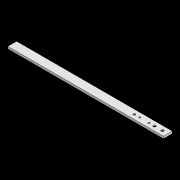
# Autodesk Inventor part: arm1_L
Saved by Autodesk Inventor 2022 (Build 260153000, 153)
## iProperties
Created: 2021-06-08
Part Number: arm1_L
Material: 一般
Document SubType Name: Modeling
Designer: yossy
Density: 1 g/cm^3
Appearance: 既定
Mass: 42.0818 g
Surface Area: 203.017 cm^2
Volume: 15.5858 cm^3
Author: yossy
Autodesk Inventor part; units mm, degrees
ref_plane "YZ Plane" through (0, 0, 0) normal (1, 0, 0) x (0, 1, 0)
ref_plane "XZ Plane" through (0, 0, 0) normal (0, 1, 0) x (-1, 0, 0)
ref_plane "XY Plane" through (0, 0, 0) normal (0, 0, 1) x (1, 0, 0)
sketch "スケッチ1" plane through (0, 0, 0) normal (0, 0, 1) x (1, 0, 0)
  line L0 (0, 0) -> (352, 0)
  line L1 (352, 0) -> (352, 5)
  line L2 (352, 5) -> (0, 5)
  line L3 (0, 5) -> (0, 0)
  line L4 (0, 0) -> (6, 0)
  line L5 (0, 1) -> (0, 0)
  dimension "d0" = 352
  dimension "d1" = 5
  constraints: 12 end point, 2 horizontal, 2 parallel, 1 perpendicular
  measures "d0" distance of L2.end L1.end
  measures "d1" distance of L1.end L0.end
extrude "押し出し1" add sketch "スケッチ1" along normal blind 20
sketch "スケッチ3" plane through (0, 0, 0) normal (-1, 0, 0) x (0, 0, 1)
  line L0 (0, 5) -> (0, 0) projected
  line L1 (0, 0) -> (20, 0) projected
  line L2 (20, 5) -> (20, 0) projected
  line L3 (0, 5) -> (20, 5) projected
  circle A0 centre (4, 2) radius 1.2
  circle A1 centre (16, 3) radius 1.2
  dimension "d14" = 2.4
  dimension "d15" = 2.4
  dimension "d16" = 3
  dimension "d17" = 4
  dimension "d18" = 4
  dimension "d19" = 3
  constraints: 2 centre point
  measures "d14" diameter of A0
  measures "d15" diameter of A1
  measures "d16" distance from line of L1 A1.centre
  measures "d17" distance from line of L2 A1.centre
  measures "d18" distance from line of L0 A0.centre
  measures "d19" distance from line of L3 A0.centre
extrude "押し出し3" cut sketch "スケッチ3" against normal blind 6 contours A0 | A1
sketch "スケッチ4" plane through (0, 0, 0) normal (0, -1, 0) x (1, 0, 0)
  line L0 (0, 0) -> (352, 0) projected
  line L1 (352, 0) -> (352, 20) projected
  line L2 (0, 20) -> (352, 20) projected
  line L3 (0, 0) -> (0, 20) projected
  line L4 (2, 2) -> (350, 2)
  line L5 (350, 2) -> (350, 18)
  line L6 (350, 18) -> (2, 18)
  line L7 (2, 18) -> (2, 2)
  dimension "d22" = 2
  dimension "d23" = 2
  dimension "d24" = 2
  dimension "d25" = 2
  constraints: 8 end point, 2 parallel, 1 horizontal, 1 perpendicular
  measures "d22" distance between parallel lines of L3 L7
  measures "d23" distance between parallel lines of L2 L6
  measures "d24" distance between parallel lines of L0 L4
  measures "d25" distance between parallel lines of L1 L5
extrude "押し出し4" cut sketch "スケッチ4" against normal blind 3 contours L7 L6 L5 L4
sketch "スケッチ6" plane through (0, 3, 0) normal (0, -1, 0) x (1, 0, 0)
  line L0 (350, 18) -> (350, 2) projected
  line L1 (2, 18) -> (350, 18) projected
  point P0 (0, 0)
  point P1 (340, 10)
  dimension "d35" = 10
  dimension "d36" = 8
  dimension "d37" = 16
  measures "d35" distance from line of L0 point (340, 10)
  measures "d36" distance from line of L1 point (340, 10)
  measures "d37" distance of L0.start L0.end
hole "穴1" at (340, 3, 10) direction (0, 1, 0) diameter 10 end through all
sketch "スケッチ7" plane through (0, 3, 0) normal (0, -1, 0) x (1, 0, 0)
  circle A0 centre (340, 10) radius 5 projected
  line L0 (340, 10) -> (322, 10)
  point P0 (0, 0)
  dimension "d38" = 18
  constraints: 2 end point, 1 horizontal
  measures "d38" distance of L0.start L0.end
hole "穴2" at (322, 3, 10) direction (0, 1, 0) diameter 6 end through all
sketch "スケッチ8" plane through (0, 3, 0) normal (0, -1, 0) x (1, 0, 0)
  circle A0 centre (322, 10) radius 3 projected
  line L0 (322, 10) -> (309.5, 10)
  point P0 (0, 0)
  dimension "d46" = 12.5
  constraints: 2 end point, 1 horizontal
  measures "d46" distance of L0.start L0.end
hole "穴3" at (309.5, 3, 10) direction (0, 1, 0) diameter 7 end through all
sketch "スケッチ9" plane through (0, 3, 0) normal (0, -1, 0) x (1, 0, 0)
  circle A0 centre (309.5, 10) radius 3.5 projected
  line L0 (309.5, 10) -> (288.5, 10)
  point P0 (0, 0)
  dimension "d54" = 21
  constraints: 2 end point, 1 horizontal
  measures "d54" distance of L0.start L0.end
hole "穴4" at (288.5, 3, 10) direction (0, 1, 0) diameter 7 end through all
sketch "スケッチ10" plane through (0, 3, 0) normal (0, -1, 0) x (1, 0, 0)
  circle A0 centre (288.5, 10) radius 3.5 projected
  line L0 (288.5, 10) -> (276.5, 10)
  point P0 (0, 0)
  dimension "d62" = 12
  constraints: 2 end point, 1 horizontal
  measures "d62" distance of L0.start L0.end
hole "穴5" at (276.5, 3, 10) direction (0, 1, 0) diameter 7 end through all
equation "\"d36\" = 0.5 * d37"
